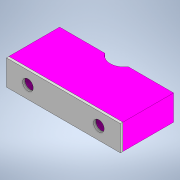
# Autodesk Inventor part: hull_rudder_tube_clamp
Saved by Autodesk Inventor 2020 (Build 240168000, 168)
## iProperties
Created: 2019-11-18
Part Number: hull_rudder_tube_clamp
Material: Generic
Document SubType Name: Modeling
Designer: suchanek
Density: 1 g/cm^3
Appearance: Default
Author: suchanek
Autodesk Inventor part; units mm, degrees
ref_plane "YZ Plane" through (0, 0, 0) normal (1, 0, 0) x (0, 1, 0)
ref_plane "XZ Plane" through (0, 0, 0) normal (0, 1, 0) x (-1, 0, 0)
ref_plane "XY Plane" through (0, 0, 0) normal (0, 0, 1) x (1, 0, 0)
sketch "Sketch1" plane through (0, 0, 0) normal (0, 1, 0) x (-1, 0, 0)
  line L0 (22.5, 0) -> (-22.5, 0)
  line L1 (-22.5, 0) -> (-22.5, 20)
  line L2 (-22.5, 20) -> (22.5, 20)
  line L3 (22.5, 20) -> (22.5, 0)
  arc A0 (4.6098, 0) -> (-4.6098, 0) centre (0, -3) ccw
  point P0 (0, 0)
  point P1 (0, 0)
  dimension "d0" = 45
  dimension "d1" = 20
  dimension "d2" = 5.5
  dimension "d3" = 3
  constraints: 8 end point, 2 parallel, 2 point on circle, 2 point on line, 1 centre point, 1 coincident, 1 horizontal, 1 midpoint, 1 perpendicular, 1 vertical alignment
  measures "d0" distance of L1.end L2.end
  measures "d1" distance of L0.end L1.end
  measures "d2" radius of A0
  measures "d3" distance of point (0, 0) A0.centre
extrude "Extrusion1" add sketch "Sketch1" along normal blind 10 contours L0 A0 L1 L2 L3
sketch "Sketch2" plane through (-22.5, 0, 20) normal (0, 0, 1) x (1, 0, 0)
  circle A0 centre (8.5, 5) radius 2.1
  line L0 (22.5, 0) -> (22.5, 4.9707)
  circle A1 centre (36.5, 5) radius 2.1
  line L1 (0, 0) -> (0, 10) projected
  line L2 (0, 0) -> (45, 0) projected
  dimension "d6" = 4.2
  dimension "d7" = 8.5
  dimension "d8" = 5
  constraints: 2 centre point, 2 end point, 1 symmetric about line, 1 vertical, 1 other
  measures "d6" diameter of A0
  measures "d7" distance from line of L1 A0.centre
  measures "d8" distance from line of L2 A0.centre
extrude "Extrusion2" cut sketch "Sketch2" against normal through all
sketch "Sketch3" plane through (-22.5, 0, 20) normal (0, 0, 1) x (1, 0, 0)
  line L0 (17.8902, 0) -> (0, 0) projected
  line L1 (45, 10) -> (27.1098, 10) projected
  line L2 (0, 0) -> (45, 0)
  line L3 (45, 0) -> (45, 10)
  line L4 (45, 10) -> (0, 10)
  line L5 (0, 10) -> (0, 0)
  circle A0 centre (8.5, 5) radius 2.1 projected
  circle A1 centre (8.5, 5) radius 2.1
  circle A2 centre (36.5, 5) radius 2.1 projected
  circle A3 centre (36.5, 5) radius 2.1
  point P0 (22.5, 0)
  constraints: 8 end point, 2 centre point, 2 coincident, 2 parallel, 1 horizontal, 1 perpendicular
extrude "Extrusion3" add sketch "Sketch3" along normal blind 1 separate body
body "Solid1"
body "Solid2"
